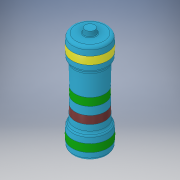
# Autodesk Inventor part: HVU_resistor_5M1_(VR25000005104JA100)
Saved by Autodesk Inventor 2017 (Build 210142000, 142)
## iProperties
Part Number: HVU_resistor_5M1_(VR25000005104JA100)
Material: Generisch
Document SubType Name: Modeling
Designer: Philomena-Theresa
Density: 1 g/cm^3
Appearance: Türkis
Author: Philomena-Theresa
Autodesk Inventor part; units mm, degrees
ref_plane "YZ Plane" through (0, 0, 0) normal (1, 0, 0) x (0, 1, 0)
ref_plane "XZ Plane" through (0, 0, 0) normal (0, 1, 0) x (-1, 0, 0)
ref_plane "XY Plane" through (0, 0, 0) normal (0, 0, 1) x (1, 0, 0)
sketch "Skizze5" plane through (0, 0, 0) normal (0, 1, 0) x (-1, 0, 0)
  line L0 (0, 4.4678) -> (0, 0)
  line L1 (0.95, 0) -> (0, 0)
  line L2 (0.4, 3.2) -> (0.9115, 3.2)
  line L3 (0.9115, 1.7) -> (0.4352, 1.7) construction
  arc A0 (1.1096, 3.0278) -> (0.9115, 3.2) centre (0.9115, 3) ccw
  arc A1 (0.9115, 1.7) -> (1.0559, 1.7615) centre (0.9115, 1.9) ccw construction
  arc A2 (1.1096, 1.8722) -> (1.1096, 3.0278) centre (-3.0019, 2.45) ccw
  line L4 (1.15, 2.45) -> (-3.0019, 2.45) construction
  line L5 (0.9115, 1.9) -> (0.9115, 3) construction
  arc A3 (1.0559, 1.7615) -> (1.1096, 1.8722) centre (0.9115, 1.9) ccw
  arc A4 (0.3542, 3.23) -> (0.4, 3.2) centre (0.4, 3.25) ccw
  line L6 (0.9115, 3) -> (1.1096, 3.0278) construction
  arc A5 (1.0559, 1.7615) -> (0.9889, 1.6061) centre (1.2301, 1.5944) ccw
  line L7 (0.3, 3.5) -> (0, 3.5)
  line L8 (0, 3.5) -> (0, 0)
  arc A6 (0.3, 3.5) -> (0.3542, 3.23) centre (0.9523, 3.4904) ccw
  arc A7 (0.9889, 1.6061) -> (0.95, 0) centre (34.092, 0) ccw
  line L9 (34.092, 0) -> (0.95, 0) construction
  dimension "d12" = 1.5
  dimension "d14" = 0.2
  dimension "d16" = 1.9
  dimension "d17" = 2.3
  dimension "d18" = 0.75
  dimension "d21" = 98
  dimension "d22" = 0.3
  dimension "d23" = 3.2
  constraints: 20 end point, 17 point on circle, 9 tangent, 8 centre point, 3 horizontal, 2 vertical, 1 collinear, 1 perpendicular, 1 point on line
  measures "d12" distance between parallel lines of L2 L3
  measures "d14" radius of A0
  measures "d16" diameter of L1.start L0
  measures "d17" diameter of L4.start L0
  measures "d18" distance between parallel lines of L2 L4
  measures "d21" angle of L5 L6
  measures "d22" distance between parallel lines of L2 L7
  measures "d23" distance between parallel lines of L2 L1
revolve "Umdrehung1" add sketch "Skizze5" angle 360 about axis through (0, 0, 4.4678) along (0, 0, -1)
mirror "Spiegeln2" about plane through (0, 0, 0) normal (0, 0, 1) of "Umdrehung1"
sketch "Skizze6" plane through (0, 0, 0) normal (0, 1, 0) x (-1, 0, 0)
  arc A0 (1.1096, 1.8722) -> (1.1096, 3.0278) centre (-3.0019, 2.45) ccw projected
  arc A1 (1.1425, 2.2) -> (1.1425, 2.7) centre (-1.3446, 2.45) ccw
  line L0 (-3.0019, 2.45) -> (-1.3446, 2.45)
  line L1 (0, -4.9) -> (0, 4.9) projected
  point P0 (0, 0)
  dimension "d25" = 0.5
  dimension "d26" = 0.005
  constraints: 4 point on circle, 2 end point, 1 centre point, 1 horizontal
  measures "d25" distance of A1.end A1.start
revolve "Umdrehung2" add sketch "Skizze6" angle 360 about axis through (0, 0, -10) along (0, 0, 1)
mirror "Spiegeln3" about plane through (0, 0, 0) normal (0, 0, 1) of "Umdrehung2"
sketch "Skizze7" plane through (0, 0, 0) normal (0, 1, 0) x (-1, 0, 0)
  arc A0 (0.9889, 1.6061) -> (0.9889, -1.6061) centre (34.092, 0) ccw projected
  arc A1 (0.9509, -0.25) -> (0.9509, 0.25) centre (-6.7496, 0) ccw
  line L0 (-6.7496, 0) -> (0, 0)
  line L1 (0.9509, 0.25) -> (0.9509, -0.25) construction
  line L2 (0, -4.9) -> (0, 4.9) projected
  dimension "d28" = 0.005
  dimension "d29" = 0.5
  constraints: 4 end point, 4 point on circle, 1 centre point, 1 horizontal
  measures "d29" distance of L1.start L1.end
revolve "Umdrehung3" add sketch "Skizze7" angle 360 about axis through (0, 0, -10) along (0, 0, 1)
sketch "Skizze8" plane through (0, 0, 0) normal (0, 1, 0) x (-1, 0, 0)
  arc A0 (0.9509, -0.25) -> (0.9889, -1.6061) centre (34.092, 0) ccw projected
  line L0 (0, 0) -> (-1.7052, 0)
  line L1 (-6.731, -1.2322) -> (0.235, -1.2322)
  arc A1 (0.9736, -1.2498) -> (0.9585, -0.75) centre (-6.731, -1.2322) ccw
  line L2 (0.9736, -1.2498) -> (0.9585, -0.75) construction
  line L3 (0, -4.9) -> (0, 4.9) projected
  dimension "d32" = 0.005
  dimension "d34" = 0.5
  dimension "d35" = 0.5
  constraints: 6 end point, 4 point on circle, 2 horizontal, 1 centre point, 1 coincident
  measures "d34" distance of L2.start L2.end
  measures "d35" vertical distance of A0.start L2.end
revolve "Umdrehung4" add sketch "Skizze8" angle 360 about axis through (0, 0, -10) along (0, 0, 1)
equation "\"d18\" = 0.5 * d12"
